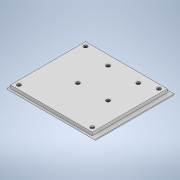
# Autodesk Inventor part: Electronics Box Lid
Saved by Autodesk Inventor 2022 (Build 260153000, 153)
## iProperties
Created: 2021-09-21
Part Number: Electronics Box Lid
Material: Generic
Document SubType Name: Modeling
Designer: kylem
Density: 1 g/cm^3
Appearance: Default
Author: kylem
Autodesk Inventor part; units mm, degrees
ref_plane "YZ Plane" through (0, 0, 0) normal (1, 0, 0) x (0, 1, 0)
ref_plane "XZ Plane" through (0, 0, 0) normal (0, 1, 0) x (-1, 0, 0)
ref_plane "XY Plane" through (0, 0, 0) normal (0, 0, 1) x (1, 0, 0)
sketch "Sketch1" plane through (0, 0, 0) normal (0, 1, 0) x (-1, 0, 0)
  line L0 (0, 0) -> (82, 0)
  line L1 (82, 0) -> (82, -73.75)
  line L2 (82, -73.75) -> (0, -73.75)
  line L3 (0, -73.75) -> (0, 0)
  dimension "d0" = 82
  dimension "d1" = 73.75
  constraints: 8 end point, 2 parallel, 1 horizontal, 1 perpendicular
  measures "d0" distance of L1.end L2.end
  measures "d1" distance of L0.end L1.end
extrude "Extrusion1" add sketch "Sketch1" along normal blind 1
sketch "Sketch2" plane through (0, 1, 0) normal (0, 1, 0) x (1, 0, 0)
  line L0 (-82, 0) -> (0, 0) projected
  line L1 (0, 0) -> (-4, 0)
  line L2 (-4, 0) -> (-4, 2)
  line L3 (-4, 2) -> (0, 2)
  line L4 (0, 2) -> (0, 0)
  line L5 (0, 73.75) -> (-82, 73.75) projected
  line L6 (0, 73.75) -> (-4, 73.75)
  line L7 (-4, 73.75) -> (-4, 71.75)
  line L8 (-4, 71.75) -> (0, 71.75)
  line L9 (0, 71.75) -> (0, 73.75)
  line L10 (0, 73.75) -> (-82, 73.75)
  line L11 (-82, 0) -> (-80, 0)
  line L12 (-80, 0) -> (-80, 2)
  line L13 (-80, 2) -> (-82, 2)
  line L14 (-82, 2) -> (-82, 0)
  line L15 (-82, 73.75) -> (-82, 0) projected
  line L16 (-82, 73.75) -> (-80, 73.75)
  line L17 (-80, 73.75) -> (-80, 71.75)
  line L18 (-80, 71.75) -> (-82, 71.75)
  line L19 (-82, 71.75) -> (-82, 73.75)
  line L20 (-4, 2) -> (-80, 2)
  line L21 (-80, 2) -> (-80, 71.75)
  line L22 (-80, 71.75) -> (-4, 71.75)
  line L23 (-4, 71.75) -> (-4, 2)
  dimension "d4" = 4
  dimension "d5" = 2
  dimension "d6" = 4
  dimension "d7" = 2
  dimension "d8" = 2
  dimension "d9" = 2
  dimension "d10" = 2
  dimension "d11" = 2
  constraints: 42 end point, 11 equal length, 5 horizontal, 5 perpendicular
  measures "d4" distance of L2.end L3.end
  measures "d5" distance of L1.end L2.end
  measures "d6" distance of L8.end L7.end
  measures "d7" distance of L7.end L6.end
  measures "d8" distance of L13.end L12.end
  measures "d9" distance of L12.end L11.end
  measures "d10" distance of L17.end L18.end
  measures "d11" distance of L16.end L17.end
extrude "Extrusion2" add sketch "Sketch2" along normal blind 3 contours L21 L22 L23 L20
sketch "Sketch3" plane through (0, 0, 0) normal (0, -1, 0) x (1, 0, 0)
  line L0 (-82, -73.75) -> (-82, 0) projected
  line L1 (-82, -73.75) -> (-50.14, -73.75)
  line L2 (-50.14, -73.75) -> (-50.14, -62.75)
  line L3 (-50.14, -62.75) -> (-82, -62.75)
  line L4 (-82, -62.75) -> (-82, -73.75)
  line L5 (-50.14, -62.75) -> (-22.14, -62.75)
  line L6 (-22.14, -62.75) -> (-22.14, -34.75)
  line L7 (-22.14, -34.75) -> (-50.14, -34.75)
  line L8 (-50.14, -34.75) -> (-50.14, -62.75)
  circle A0 centre (-22.14, -62.75) radius 1.75
  circle A1 centre (-22.14, -34.75) radius 1.75
  circle A2 centre (-50.14, -34.75) radius 1.75
  circle A3 centre (-50.14, -62.75) radius 1.75
  point P0 (0, 0)
  point P1 (-48.39, -62.75)
  point P2 (-50.14, -61)
  point P3 (-51.89, -62.75)
  point P4 (-50.14, -64.5)
  point P5 (-23.89, -62.75)
  point P6 (-22.14, -61)
  point P7 (-22.14, -36.5)
  point P8 (-23.89, -34.75)
  point P9 (-48.39, -34.75)
  point P10 (-50.14, -36.5)
  dimension "d14" = 31.86
  dimension "d15" = 11
  dimension "d16" = 28
  dimension "d17" = 28
  dimension "d18" = 3.5
  dimension "d19" = 3.5
  dimension "d20" = 3.5
  dimension "d21" = 3.5
  constraints: 16 end point, 4 centre point, 4 coincident, 4 parallel, 2 horizontal, 2 perpendicular
  measures "d14" distance of L3.end L2.end
  measures "d15" distance of L2.end L1.end
  measures "d16" distance of L7.end L6.end
  measures "d17" distance of L6.end L5.end
  measures "d18" diameter of A0
  measures "d19" diameter of A1
  measures "d20" diameter of A2
  measures "d21" diameter of A3
extrude "Extrusion3" cut sketch "Sketch3" against normal blind 5 contours A3 L8 L3 | L3 L2 A3 | L2 L5 A3 | L8 A3 L5 | A2 L7 L8 | L8 L7 A2 | A0 L6 L5 | L5 L6 A0 | A1 L6 L7 | L7 L6 A1
sketch "Sketch4" plane through (0, 0, 0) normal (0, -1, 0) x (1, 0, 0)
  circle A0 centre (-22.14, -62.75) radius 1.75 projected
  circle A1 centre (-22.14, -62.75) radius 3.25
  circle A2 centre (-50.14, -62.75) radius 1.75 projected
  circle A3 centre (-50.14, -62.75) radius 3.25
  circle A4 centre (-50.14, -34.75) radius 1.75 projected
  circle A5 centre (-50.14, -34.75) radius 3.25
  circle A6 centre (-22.14, -34.75) radius 1.75 projected
  circle A7 centre (-22.14, -34.75) radius 3.25
  point P0 (0, 0)
  dimension "d24" = 6.5
  dimension "d25" = 6.5
  dimension "d26" = 6.5
  dimension "d27" = 6.5
  constraints: 4 centre point, 4 coincident
  measures "d24" diameter of A1
  measures "d25" diameter of A3
  measures "d26" diameter of A5
  measures "d27" diameter of A7
extrude "Extrusion4" cut sketch "Sketch4" against normal blind 3
sketch "Sketch5" plane through (0, 4, 0) normal (0, 1, 0) x (1, 0, 0)
  line L0 (-4, 71.75) -> (-80, 71.75) projected
  line L1 (-80, 71.75) -> (-76, 71.75)
  line L2 (-80, 71.75) -> (-76, 71.75)
  line L3 (-76, 71.75) -> (-76, 67.75)
  line L4 (-76, 67.75) -> (-80, 67.75)
  line L5 (-80, 67.75) -> (-80, 71.75)
  line L6 (-4, 71.75) -> (-8, 71.75)
  line L7 (-8, 71.75) -> (-8, 67.75)
  line L8 (-8, 67.75) -> (-4, 67.75)
  line L9 (-4, 67.75) -> (-4, 71.75)
  line L10 (-80, 2) -> (-4, 2) projected
  line L11 (-4, 2) -> (-8, 2)
  line L12 (-8, 2) -> (-8, 6)
  line L13 (-8, 6) -> (-4, 6)
  line L14 (-4, 6) -> (-4, 2)
  line L15 (-80, 2) -> (-76, 2)
  line L16 (-76, 2) -> (-76, 6)
  line L17 (-76, 6) -> (-80, 6)
  line L18 (-80, 6) -> (-80, 2)
  circle A0 centre (-76, 67.75) radius 1.75
  circle A1 centre (-8, 67.75) radius 1.75
  circle A2 centre (-8, 6) radius 1.75
  circle A3 centre (-76, 6) radius 1.75
  point P0 (0, 0)
  dimension "d30" = 4
  dimension "d31" = 4
  dimension "d32" = 4
  dimension "d33" = 4
  dimension "d34" = 4
  dimension "d35" = 4
  dimension "d36" = 4
  dimension "d37" = 4
  dimension "d38" = 4
  dimension "d39" = 3.5
  dimension "d40" = 3.5
  dimension "d41" = 3.5
  dimension "d42" = 3.5
  constraints: 34 end point, 8 parallel, 4 centre point, 4 coincident, 4 horizontal, 4 perpendicular, 3 point on line
  measures "d30" distance of L0.end L1.end
  measures "d31" distance of L3.end L4.end
  measures "d32" distance of L2.end L3.end
  measures "d33" distance of L8.end L7.end
  measures "d34" distance of L7.end L6.end
  measures "d35" distance of L12.end L13.end
  measures "d36" distance of L11.end L12.end
  measures "d37" distance of L17.end L16.end
  measures "d38" distance of L16.end L15.end
  measures "d39" diameter of A0
  measures "d40" diameter of A1
  measures "d41" diameter of A2
  measures "d42" diameter of A3
extrude "Extrusion5" cut sketch "Sketch5" against normal blind 5 contours A1 L8 L7 | L7 L8 A1 | A0 L4 L3 | L3 L4 A0 | A3 L17 L16 | L16 L17 A3 | A2 L13 L12 | L12 L13 A2
sketch "Sketch6" plane through (0, 0, 0) normal (0, -1, 0) x (1, 0, 0)
  circle A0 centre (-8, -67.75) radius 1.75 projected
  circle A1 centre (-8, -67.75) radius 3.25
  circle A2 centre (-76, -67.75) radius 1.75 projected
  circle A3 centre (-76, -67.75) radius 3.25
  circle A4 centre (-76, -6) radius 1.75 projected
  circle A5 centre (-76, -6) radius 3.25
  circle A6 centre (-8, -6) radius 1.75 projected
  circle A7 centre (-8, -6) radius 3.25
  point P0 (0, 0)
  dimension "d45" = 6.5
  dimension "d46" = 6.5
  dimension "d47" = 6.5
  dimension "d48" = 6.5
  constraints: 4 centre point, 4 coincident
  measures "d45" diameter of A1
  measures "d46" diameter of A3
  measures "d47" diameter of A5
  measures "d48" diameter of A7
extrude "Extrusion6" cut sketch "Sketch6" against normal blind 3 contours A0 | A1 | A2 | A3 | A4 | A5 | A6 | A7
sketch "Sketch7" plane through (0, 4, 0) normal (0, 1, 0) x (1, 0, 0)
  line L0 (-4, 2) -> (-4, 71.75) projected
  line L1 (-4, 2) -> (-4.12, 2)
  line L2 (-4.12, 2) -> (-4.12, 2.12)
  line L3 (-4.12, 2.12) -> (-4, 2.12)
  line L4 (-4, 2.12) -> (-4, 2)
  line L5 (-80, 71.75) -> (-4, 71.75) projected
  line L6 (-80, 71.75) -> (-79.88, 71.75)
  line L7 (-79.88, 71.75) -> (-79.88, 71.63)
  line L8 (-79.88, 71.63) -> (-80, 71.63)
  line L9 (-80, 71.63) -> (-80, 71.75)
  line L10 (-79.88, 71.63) -> (-4, 71.63)
  line L11 (-4, 71.63) -> (-4, 71.75)
  line L12 (-4, 71.75) -> (-79.88, 71.75)
  line L13 (-79.88, 71.75) -> (-79.88, 71.63)
  line L14 (-4.12, 2) -> (-4, 2)
  line L15 (-4, 2) -> (-4, 71.75)
  line L16 (-4, 71.75) -> (-4.12, 71.75)
  line L17 (-4.12, 71.75) -> (-4.12, 2)
  line L18 (-80, 2) -> (-4, 2) projected
  line L19 (-4.12, 2.12) -> (-80, 2.12)
  line L20 (-80, 2.12) -> (-80, 2)
  line L21 (-80, 2) -> (-4.12, 2)
  line L22 (-4.12, 2) -> (-4.12, 2.12)
  line L23 (-80, 2) -> (-79.88, 2)
  line L24 (-79.88, 2) -> (-79.88, 71.63)
  line L25 (-79.88, 71.63) -> (-80, 71.63)
  line L26 (-80, 71.63) -> (-80, 2)
  point P0 (0, 0)
  point P1 (-4.12, 2.12)
  point P2 (-79.88, 2.12)
  point P3 (-4.12, 71.63)
  dimension "d51" = 0.12
  dimension "d52" = 0.12
  dimension "d53" = 0.12
  dimension "d54" = 0.12
  constraints: 48 end point, 12 parallel, 6 horizontal, 6 perpendicular, 2 point on line
  measures "d51" distance of L2.end L3.end
  measures "d52" distance of L1.end L2.end
  measures "d53" distance of L7.end L8.end
  measures "d54" distance of L6.end L7.end
extrude "Extrusion7" cut sketch "Sketch7" against normal blind 3 contours L1 L2 L3 L0 | L3 L17 L10 L0 | L18 L24 L19 L2 | L10 L17 L5 L0 | L18 L20 L19 L24 | L10 L7 L5 L17 | L19 L26 L8 L24 | L8 L9 L5 L7
chamfer "Chamfer1" distance 1 angle 45 3 edges at (-41, 0, -73.75) (-82, 0, -36.875) (-41, 0, 0)
chamfer "Chamfer2" distance 1 angle 45 2 edges at (-81.5001, 0.4999, -73.2501) (-81.5001, 0.4999, -0.4999)
body "Solid1"
